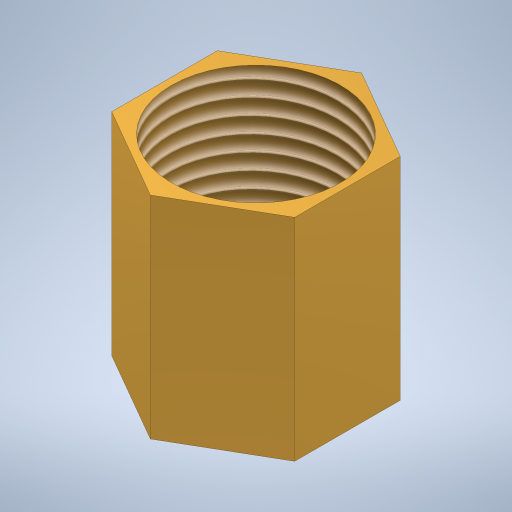
# Autodesk Inventor part: Pieza 1 subensamble 1-69
Saved by Autodesk Inventor 2024.2 (Build 282272000, 272)
## iProperties
Created: 2024-11-02
Part Number: Pieza 1 subensamble 1-69
Material: Latón, amarillo claro
Document SubType Name: Modeling
Designer: Monica Mora
Density: 8.47 g/cm^3
Appearance: Latón - Satinado
Author: Monica Mora
Autodesk Inventor part; units mm, degrees
ref_plane "YZ Plane" through (0, 0, 0) normal (1, 0, 0) x (0, 1, 0)
ref_plane "XZ Plane" through (0, 0, 0) normal (0, 1, 0) x (-1, 0, 0)
ref_plane "XY Plane" through (0, 0, 0) normal (0, 0, 1) x (1, 0, 0)
sketch "Boceto1" plane through (0, 0, 0) normal (0, 1, 0) x (-1, 0, 0)
  line L0 (0, 5) -> (4.3301, 2.5)
  line L1 (4.3301, 2.5) -> (4.3301, -2.5)
  line L2 (4.3301, -2.5) -> (0, -5)
  line L3 (0, -5) -> (-4.3301, -2.5)
  line L4 (-4.3301, -2.5) -> (-4.3301, 2.5)
  line L5 (-4.3301, 2.5) -> (0, 5)
  circle A0 centre (0, 0) radius 4
  circle A1 centre (0, 0) radius 2
  dimension "d0" = 10
  dimension "d1" = 8
  dimension "d2" = 4
  constraints: 12 end point, 3 coincident, 2 centre point, 13 other
  measures "d0" distance of L0.start L2.end
  measures "d1" diameter of A0
  measures "d2" diameter of A1
extrude "Extrusión1" add sketch "Boceto1" along normal blind 10 contours L0 L1 L2 L3 L4 L5
extrude "Extrusión2" add sketch "Boceto1" along normal blind 2 contours A0
thread "Rosca1" size "M8x0.75" class "6H" standard "ANSI Metric M Profile" length 6
